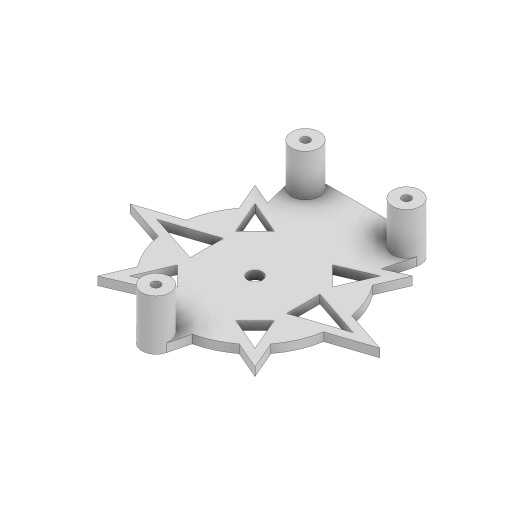
# Autodesk Inventor part: BASE_LIDAR_V2
Saved by Autodesk Inventor 2024.2 (Build 282272000, 272)
## iProperties
Created: 2024-07-17
Part Number: BASE_LIDAR_V2
Material: Generic
Document SubType Name: Modeling
Designer: jrcer
Density: 1 g/cm^3
Appearance: Default
Author: jrcer
Autodesk Inventor part; units mm, degrees
ref_plane "YZ Plane" through (0, 0, 0) normal (1, 0, 0) x (0, 1, 0)
ref_plane "XZ Plane" through (0, 0, 0) normal (0, 1, 0) x (-1, 0, 0)
ref_plane "XY Plane" through (0, 0, 0) normal (0, 0, 1) x (1, 0, 0)
sketch "Sketch1" plane through (0, 0, 0) normal (0, 1, 0) x (-1, 0, 0)
  circle A0 centre (0, 35.3) radius 1.55
  circle A1 centre (18, -36) radius 1.55
  circle A2 centre (-18, -36) radius 1.55
  circle A3 centre (0, 35.3) radius 5
  circle A4 centre (18, -36) radius 5
  circle A5 centre (-18, -36) radius 5
  point P0 (0, 0)
  dimension "d0" = 35.3
  dimension "d1" = 36
  dimension "d2" = 3.1
  dimension "d3" = 10
  dimension "d4" = 36
  dimension "d5" = 18
  constraints: 6 centre point, 4 equal radius, 3 coincident, 1 horizontal alignment, 1 vertical alignment
  measures "d0" distance of A0.centre point (0, 0)
  measures "d1" vertical distance of A2.centre point (0, 0)
  measures "d2" diameter of A0
  measures "d3" diameter of A3
  measures "d4" distance of A2.centre A1.centre
  measures "d5" horizontal distance of point (0, 0) A2.centre
extrude "Extrusion1" add sketch "Sketch1" along normal blind 15
sketch "Sketch2" plane through (0, 0, 35.3) normal (0, -1, 0) x (1, 0, 0)
  circle A0 centre (0, 0) radius 5 projected
  circle A1 centre (0, 0) radius 1.55 projected
  circle A2 centre (-18, -71.3) radius 1.55 projected
  circle A3 centre (-18, -71.3) radius 5 projected
  circle A4 centre (18, -71.3) radius 1.55 projected
  circle A5 centre (18, -71.3) radius 5 projected
  line L0 (-22.8479, -70.0761) -> (-4.8479, 1.2239)
  line L1 (22.8479, -70.0761) -> (4.8479, 1.2239)
  line L2 (-18, -76.3) -> (18, -76.3)
  circle A6 centre (0, -35.3) radius 2.6
  dimension "d8" = 5.2
  constraints: 6 end point, 6 point on circle, 5 tangent, 1 centre point, 1 coincident, 1 horizontal
  measures "d8" diameter of A6
extrude "Extrusion2" add sketch "Sketch2" along normal blind 3
sketch "Sketch6" plane through (0, -3, 35.3) normal (0, -1, 0) x (1, 0, 0)
  circle A0 centre (0, -35.3) radius 2.6 projected
  circle A1 centre (0, -35.3) radius 29.9
  line L0 (22.8479, -70.0761) -> (4.8479, 1.2239) projected
  line L1 (-4.8479, 1.2239) -> (-22.8479, -70.0761) projected
  point P0 (-19.7384, -57.759)
  point P1 (-6.7128, -6.1633)
  point P2 (6.7128, -6.1633)
  point P3 (19.7384, -57.759)
  dimension "d41" = 59.8
  constraints: 1 centre point, 1 coincident
  measures "d41" diameter of A1
extrude "Extrusion6" add sketch "Sketch6" against normal blind 3 contours A1 L0 | L1 A1
sketch "Sketch7" plane through (0, 0, 35.3) normal (0, 1, 0) x (1, 0, 0)
  arc A0 (-19.7384, 57.759) -> (-6.7128, 6.1633) centre (0, 35.3) ccw projected
  arc A1 (6.7128, 6.1633) -> (19.7384, 57.759) centre (0, 35.3) ccw projected
  circle A2 centre (0, 35.3) radius 29.9 construction
  line L0 (-29.9, 35.3) -> (29.9, 35.3) construction
  line L1 (0, 5.4) -> (0, 65.2) construction
  line L2 (-21.1425, 14.1575) -> (21.1425, 56.4425) construction
  line L3 (-29.479, 30.3) -> (-44.479, 35.3)
  line L4 (-44.479, 35.3) -> (-29.479, 40.3)
  line L5 (-29.479, 30.3) -> (-29.479, 40.3)
  point P0 (0, 35.3)
  point P1 (-29.479, 40.3)
  point P2 (-29.479, 30.3)
  dimension "d44" = 59.8
  dimension "d45" = 45
  dimension "d46" = 10
  dimension "d47" = 15
  constraints: 12 end point, 6 midpoint, 2 vertical, 1 coincident, 1 horizontal, 1 horizontal alignment, 10 other
  measures "d45" angle of L1 L2
  measures "d46" distance of L4.end L3.start
  measures "d47" distance from line of L5 L3.end
extrude "Extrusion7" add sketch "Sketch7" against normal blind 3 contours A0 L3 L4
sketch "Sketch8" plane through (0, 0, 35.3) normal (0, 1, 0) x (1, 0, 0)
  line L0 (-21.1425, 14.1575) -> (21.1425, 56.4425) construction
  arc A0 (-29.479, 30.3) -> (-6.7128, 6.1633) centre (0, 35.3) ccw projected
  line L1 (-18.124, 11.5191) -> (-23.7809, 17.176)
  line L2 (-23.7809, 17.176) -> (-28.0235, 7.2765)
  line L3 (-28.0235, 7.2765) -> (-18.124, 11.5191)
  line L4 (-20.9524, 14.3476) -> (-28.0235, 7.2765) construction
  dimension "d50" = 8
  dimension "d51" = 10
  constraints: 8 end point, 2 point on circle, 1 collinear, 1 midpoint, 1 point on line
  measures "d50" distance of L1.start L1.end
  measures "d51" distance from line of L1 L2.end
extrude "Extrusion8" add sketch "Sketch8" against normal blind 3 contours A0 L3 L2
pattern_circular "Circular Pattern1" count 4 over 360 about axis through (0, -10, 0) along (0, 1, 0) of "Extrusion8"
pattern_circular "Circular Pattern2" count 2 over 360 about axis through (0, -10, 0) along (0, 1, 0) of "Extrusion7"
sketch "Sketch9" plane through (0, 0, 35.3) normal (0, 1, 0) x (1, 0, 0)
  line L0 (18.124, 11.5191) -> (28.0235, 7.2765) projected
  line L1 (28.0235, 7.2765) -> (23.7809, 17.176) projected
  line L2 (19.3058, 14.2766) -> (22.3117, 12.9883)
  line L3 (22.3117, 12.9883) -> (21.0234, 15.9942)
  line L4 (19.3058, 14.2766) -> (10.4323, 18.0795)
  line L5 (10.4323, 18.0795) -> (17.2205, 24.8677)
  line L6 (17.2205, 24.8677) -> (21.0234, 15.9942)
  line L7 (18.124, 11.5191) -> (23.7809, 17.176) construction
  point P0 (0, 35.3)
  dimension "d60" = 3
  dimension "d61" = 12
  constraints: 12 end point, 2 collinear, 1 parallel, 1 other
  measures "d60" distance between parallel lines of L0 L2
  measures "d61" distance from line of L2.end L5
extrude "Extrusion9" cut sketch "Sketch9" against normal blind 3
sketch "Sketch10" plane through (0, 0, 35.3) normal (0, 1, 0) x (1, 0, 0)
  line L0 (29.479, 30.3) -> (44.479, 35.3) projected
  line L1 (44.479, 35.3) -> (29.479, 40.3) projected
  line L2 (28.5303, 37.454) -> (34.9921, 35.3)
  line L3 (34.9921, 35.3) -> (28.5303, 33.146)
  line L4 (28.5303, 33.146) -> (17.2205, 29.3761)
  line L5 (17.2205, 29.3761) -> (17.2205, 41.2239)
  line L6 (17.2205, 41.2239) -> (28.5303, 37.454)
  point P0 (0, 35.3)
  point P1 (17.2205, 24.8677)
  dimension "d64" = 3
  constraints: 10 end point, 2 collinear, 1 vertical, 1 vertical alignment, 1 other
  measures "d64" distance between parallel lines of L1 L2
extrude "Extrusion10" cut sketch "Sketch10" against normal blind 3
pattern_circular "Circular Pattern3" count 4 over 360 about axis through (0, -10, 0) along (0, 1, 0) of "Extrusion9"
pattern_circular "Circular Pattern4" count 2 over 360 about axis through (0, -10, 0) along (0, 1, 0) of "Extrusion10"
equation "\"d5\" = 0.5 * d4"
body "Solid1"
